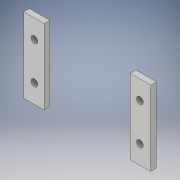
# Autodesk Inventor part: LC_mirror_holder_back
Saved by Autodesk Inventor 2019 (Build 230136000, 136)
## iProperties
Created: 2021-05-17
Part Number: LC_mirror_holder_back
Material: Generic
Document SubType Name: Modeling
Designer: UC2
Density: 1 g/cm^3
Appearance: Default
Author: UC2
Autodesk Inventor part; units mm, degrees
ref_plane "YZ Plane" through (0, 0, 0) normal (1, 0, 0) x (0, 1, 0)
ref_plane "XZ Plane" through (0, 0, 0) normal (0, 1, 0) x (-1, 0, 0)
ref_plane "XY Plane" through (0, 0, 0) normal (0, 0, 1) x (1, 0, 0)
sketch "Skizze1" plane through (0, 0, 0) normal (0, 0, 1) x (1, 0, 0)
  line L0 (-39.2, 0) -> (39.2, 0) construction
  line L1 (0, -23.1) -> (0, 23.1) construction
  line L2 (-28, -16.5) -> (28, -16.5)
  line L3 (28, -16.5) -> (28, 16.5)
  line L4 (28, 16.5) -> (-28, 16.5)
  line L5 (-28, 16.5) -> (-28, -16.5)
  line L6 (-28, -16.5) -> (28, 16.5) construction
  line L7 (28, -16.5) -> (-28, 16.5) construction
  line L8 (-19, -16.5) -> (19, -16.5)
  line L9 (19, -16.5) -> (19, 16.5)
  line L10 (19, 16.5) -> (-19, 16.5)
  line L11 (-19, 16.5) -> (-19, -16.5)
  line L12 (-19, -16.5) -> (19, 16.5) construction
  line L13 (19, -16.5) -> (-19, 16.5) construction
  line L14 (-26.75, -16.5) -> (26.75, -16.5) construction
  line L15 (26.75, -16.5) -> (26.75, 16.5) construction
  line L16 (26.75, 16.5) -> (-26.75, 16.5) construction
  line L17 (-26.75, 16.5) -> (-26.75, -16.5) construction
  line L18 (-26.75, -16.5) -> (26.75, 16.5) construction
  line L19 (26.75, -16.5) -> (-26.75, 16.5) construction
  circle A0 centre (-23.25, -8.25) radius 1.5
  circle A1 centre (23.25, -8.25) radius 1.5
  circle A2 centre (-23.25, 8.25) radius 1.5
  circle A3 centre (23.25, 8.25) radius 1.5
  point P0 (0, 0)
  dimension "d0" = 56
  dimension "d1" = 33
  dimension "d2" = 38
  dimension "d3" = 33
  dimension "d6" = 53.5
  dimension "d7" = 3
  dimension "d10" = 23.25
  dimension "d11" = 8.25
  constraints: 36 end point, 6 midpoint, 6 parallel, 4 centre point, 3 horizontal, 3 perpendicular, 3 symmetric about line, 1 point on line, 3 other
  measures "d0" distance of L3.end L4.end
  measures "d1" distance of L2.end L3.end
  measures "d2" distance of L10.end L9.end
  measures "d3" distance of L9.end L8.end
  measures "d6" distance of L16.end L15.end
  measures "d7" diameter of A0
  measures "d10" distance from line of L1 A0.centre
  measures "d11" distance from line of L14 A0.centre
extrude "Extrusion1" add sketch "Skizze1" along normal blind 2.5 contours L5 L4 L11 L2 | L9 L4 L3 L2
